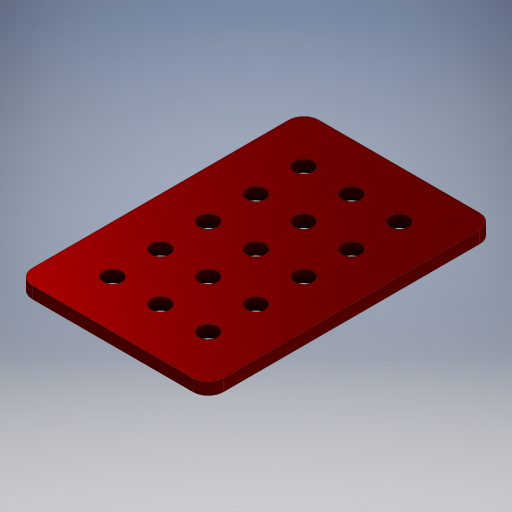
# Autodesk Inventor part: 3x5-Grid-Gusset
Saved by Autodesk Inventor 2024.2 (Build 282272000, 272)
## iProperties
Created: 2024-02-11
Part Number: 3x5-Grid-Gusset
Material: Generic
Document SubType Name: Modeling
Designer: rohan
Density: 1 g/cm^3
Appearance: Default
Author: rohan
Autodesk Inventor part; units mm, degrees
ref_plane "YZ Plane" through (0, 0, 0) normal (1, 0, 0) x (0, 1, 0)
ref_plane "XZ Plane" through (0, 0, 0) normal (0, 1, 0) x (-1, 0, 0)
ref_plane "XY Plane" through (0, 0, 0) normal (0, 0, 1) x (1, 0, 0)
sketch "Sketch1" plane through (0, 0, 0) normal (0, 1, 0) x (-1, 0, 0)
  circle A0 centre (13.0821, 0) radius 2.4892
  circle A1 centre (0.3821, 0) radius 2.4892
  line L0 (0, 10.7252) -> (0, 9.1262) construction
  circle A2 centre (-12.3179, 0) radius 2.4892
  circle A3 centre (13.0821, -12.7) radius 2.4892
  circle A4 centre (0.3821, -12.7) radius 2.4892
  circle A5 centre (-12.3179, -12.7) radius 2.4892
  circle A6 centre (13.0821, -25.4) radius 2.4892
  circle A7 centre (0.3821, -25.4) radius 2.4892
  circle A8 centre (-12.3179, -25.4) radius 2.4892
  circle A9 centre (13.0821, -38.1) radius 2.4892
  circle A10 centre (0.3821, -38.1) radius 2.4892
  circle A11 centre (-12.3179, -38.1) radius 2.4892
  circle A12 centre (13.0821, -50.8) radius 2.4892
  circle A13 centre (0.3821, -50.8) radius 2.4892
  circle A14 centre (-12.3179, -50.8) radius 2.4892
  line L1 (21.7943, 12.7) -> (-21.0301, 12.7)
  line L2 (-25.0179, 8.7122) -> (-25.0179, -59.5122)
  line L3 (-21.0301, -63.5) -> (21.7943, -63.5)
  line L4 (25.7821, -59.5122) -> (25.7821, 8.7122)
  arc A15 (25.7821, 8.7122) -> (21.7943, 12.7) centre (21.7943, 8.7122) ccw
  arc A16 (-21.0301, 12.7) -> (-25.0179, 8.7122) centre (-21.0301, 8.7122) ccw
  arc A17 (-25.0179, -59.5122) -> (-21.0301, -63.5) centre (-21.0301, -59.5122) ccw
  arc A18 (21.7943, -63.5) -> (25.7821, -59.5122) centre (21.7943, -59.5122) ccw
  point P0 (0, 0)
  point P1 (-25.0179, -63.5)
  point P2 (-25.0179, 12.7)
  point P3 (25.7821, -63.5)
  dimension "d0" = 4.9784
  dimension "d1" = 4.9784
  dimension "d2" = 12.7
  dimension "d3" = 4.9784
  dimension "d4" = 12.7
  dimension "d7" = 12.7
  dimension "d14" = 50.8
  dimension "d15" = 76.2
  dimension "d16" = 3.9878
  constraints: 19 centre point, 10 end point, 8 point on circle, 8 tangent, 6 point on line, 3 equal radius, 2 parallel, 2 vertical, 1 horizontal, 1 perpendicular, 24 other
  measures "d0" diameter of A0
  measures "d1" diameter of A1
  measures "d2" distance of A1.centre A0.centre
  measures "d3" diameter of A2
  measures "d4" distance of A1.centre A2.centre
  measures "d7" distance of A0.centre A3.centre
  measures "d14" distance of point (25.782, -63.5) point (-25.018, -63.5)
  measures "d15" distance of point (-25.018, -63.5) point (-25.018, 12.7)
  measures "d16" radius of A15
extrude "Extrusion1" add sketch "Sketch1" along normal blind 3.175
body "Solid1"
